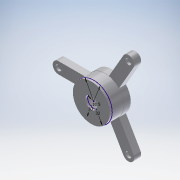
# Autodesk Inventor part: Pok Mk3 Yaw Motor Mount Mk2
Saved by Autodesk Inventor 2018.2 (Build 222227000, 227)
## iProperties
Created: 2018-02-27
Part Number: Pok Mk3 Yaw Motor Mount Mk2
Material: ABS Plastic
Document SubType Name: Modeling
Designer: Moochster
Density: 1.06 g/cm^3
Appearance: Smooth - White
Author: Moochster
Autodesk Inventor part; units mm, degrees
ref_plane "YZ Plane" through (0, 0, 0) normal (1, 0, 0) x (0, 1, 0)
ref_plane "XZ Plane" through (0, 0, 0) normal (0, 1, 0) x (-1, 0, 0)
ref_plane "XY Plane" through (0, 0, 0) normal (0, 0, 1) x (1, 0, 0)
sketch "Sketch1" plane through (0, 0, 0) normal (0, 1, 0) x (-1, 0, 0)
  circle A0 centre (0, 0) radius 15
  circle A1 centre (0, 0) radius 16.2
  line L0 (15.4091, 5) -> (40.4091, 5)
  arc A2 (40.4091, -5) -> (40.4091, 5) centre (40.4091, 0) ccw
  line L1 (40.4091, -5) -> (15.4091, -5)
  circle A3 centre (40.4091, 0) radius 2.5
  dimension "d0" = 30
  dimension "d1" = 1.2
  dimension "d2" = 5
  dimension "d3" = 25
  dimension "d4" = 5
  constraints: 4 centre point, 4 end point, 4 point on circle, 3 coincident, 2 tangent, 1 horizontal, 1 horizontal alignment, 1 parallel
  measures "d0" diameter of A0
  measures "d1" radial gap between concentric circles of A0 A1
  measures "d2" distance from line of A2.centre L1
  measures "d3" distance of L1.start L1.end
  measures "d4" diameter of A3
extrude "Extrusion1" add sketch "Sketch1" along normal blind 2 contours A1 L0 A2 L1
extrude "Extrusion2" add sketch "Sketch1" along normal blind 2 contours A1
ref_plane "Work Plane1" through (0, -10, 0) normal (0, -1, 0) x (1, 0, 0)
sketch "Sketch2" plane through (0, -10, 0) normal (0, -1, 0) x (1, 0, 0)
  circle A0 centre (0, 0) radius 5.25
  circle A1 centre (0, 0) radius 16.2
  circle A2 centre (0, 0) radius 15
  dimension "d10" = 10.5
  dimension "d12" = 30
  dimension "d22" = 1.2
  constraints: 3 centre point, 3 coincident
  measures "d10" diameter of A0
  measures "d12" diameter of A2
  measures "d22" radial gap between concentric circles of A2 A1
extrude "Extrusion3" add sketch "Sketch2" along normal blind 2 contours A1 | A2
extrude "Extrusion4" add sketch "Sketch2" against normal up to surface (10 mm away) contours A1
chamfer "Chamfer1" distance 5 angle 45 1 edges at (-16.2, 0, 0)
pattern_circular "Circular Pattern1" count 3 over 360 about axis through (0, 0, 0) along (0, 1, 0) of "Extrusion1", "Chamfer1"
sketch "Sketch4" plane through (0, 2, 0) normal (0, 1, 0) x (1, 0, 0)
  circle A0 centre (20.2045, 34.9953) radius 2.5 projected
  circle A1 centre (20.2045, -34.9953) radius 2.5 projected
  circle A2 centre (0, 0) radius 15 projected
  circle A3 centre (-40.4091, 0) radius 2.5 projected
  line L0 (-15.4091, 5) -> (-40.4091, 5) projected
  arc A4 (-40.4091, 5) -> (-40.4091, -5) centre (-40.4091, 0) ccw projected
  line L1 (-40.4091, -5) -> (-15.4091, -5) projected
  arc A5 (-15.4091, -5) -> (3.3744, -15.8447) centre (0, 0) ccw projected
  line L2 (3.3744, -15.8447) -> (15.8744, -37.4953) projected
  arc A6 (15.8744, -37.4953) -> (24.5347, -32.4953) centre (20.2045, -34.9953) ccw projected
  line L3 (24.5347, -32.4953) -> (12.0347, -10.8447) projected
  arc A7 (12.0347, -10.8447) -> (12.0347, 10.8447) centre (0, 0) ccw projected
  line L4 (12.0347, 10.8447) -> (24.5347, 32.4953) projected
  arc A8 (24.5347, 32.4953) -> (15.8744, 37.4953) centre (20.2045, 34.9953) ccw projected
  line L5 (15.8744, 37.4953) -> (3.3744, 15.8447) projected
  arc A9 (3.3744, 15.8447) -> (-15.4091, 5) centre (0, 0) ccw projected
extrude "Extrusion6" add sketch "Sketch4" along normal blind 3 contours A0 | A1 | A3 | A9 L5 A8 L4 A7 L3 A6 L2 A5 L1 A4 L0
sketch "Sketch5" plane through (0, 0, 0) normal (0, -1, 0) x (1, 0, 0)
  arc A0 (-41.1591, 4.9434) -> (-41.1591, -4.9434) centre (-40.4091, 0) ccw projected
  circle A1 centre (-40.4091, 0) radius 2.5 projected
  line L0 (-40.4091, -2.5) -> (-44.7392, -2.5)
  arc A2 (-40.4091, 5) -> (-40.4091, -5) centre (-40.4091, 0) ccw projected
  line L1 (-40.4091, 2.5) -> (-44.7392, 2.5)
  point P0 (0, 0)
  constraints: 4 end point, 4 point on circle, 2 horizontal, 2 tangent
extrude "Extrusion7" cut sketch "Sketch5" against normal blind 2 contours L1 A1 L0 A0
body "Solid1"
